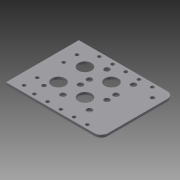
# Autodesk Inventor part: talon plate short
Saved by Autodesk Inventor 2015 (Build 190159000, 159)
## iProperties
Created: 2015-02-10
Part Number: talon plate short
Material: Generic
Document SubType Name: Modeling
Designer: sspriggs
Density: 1 g/cm^3
Appearance: Default
Mass: 12.6589 g
Surface Area: 128.442 cm^2
Volume: 12.6589 cm^3
Author: sspriggs
Autodesk Inventor part; units mm, degrees
ref_plane "YZ Plane" through (0, 0, 0) normal (1, 0, 0) x (0, 1, 0)
ref_plane "XZ Plane" through (0, 0, 0) normal (0, 1, 0) x (-1, 0, 0)
ref_plane "Work Plane1" through (-2.7575, 14.1676, 33.7809) normal (0, 1, 0) x (1, 0, 0)
sketch "Sketch1" plane through (-2.7575, 14.1676, 33.7809) normal (0, 1, 0) x (1, 0, 0)
  line L0 (-6.2522, -27.7336) -> (82.6478, -27.7336)
  line L1 (82.6478, -27.7336) -> (82.6478, -97.5836)
  line L2 (82.6478, -97.5836) -> (-6.2522, -97.5836)
  line L3 (-6.2522, -97.5836) -> (-6.2522, -27.7336)
  point P0 (2.7575, 33.7809)
  dimension "d0" = 69.85
  dimension "d1" = 88.9
  constraints: 8 end point, 2 parallel, 1 horizontal, 1 perpendicular
  measures "d0" distance of L0.end L1.end
  measures "d1" distance of L1.end L2.end
extrude "Extrusion1" add sketch "Sketch1" along normal blind 2.286
sketch "Sketch2" plane through (-2.7575, 16.4536, 33.7809) normal (0, 1, 0) x (1, 0, 0)
  line L0 (82.6478, -27.7336) -> (-6.2522, -27.7336) projected
  line L1 (-6.2522, -27.7336) -> (-6.2522, -97.5836) projected
  line L2 (-6.2522, -97.5836) -> (82.6478, -97.5836) projected
  line L3 (82.6478, -97.5836) -> (82.6478, -27.7336) projected
  circle A0 centre (5.0092, 73.556) radius 1.6383
  circle A1 centre (5.0092, 60.856) radius 1.6383
  circle A2 centre (5.0092, -2.644) radius 1.6383
  circle A3 centre (5.0092, -78.844) radius 1.6383
  circle A4 centre (5.0092, -91.544) radius 1.6383
  circle A5 centre (5.0092, -40.744) radius 1.6383
  circle A6 centre (5.0092, -53.444) radius 1.6383
  circle A7 centre (5.0092, 10.056) radius 1.6383
  constraints: 8 centre point
extrude "Extrusion2" cut sketch "Sketch2" against normal blind 2.286 contours A0 | A1 | A2 | A3 | A4 | A5 | A6 | A7
sketch "Sketch3" plane through (-2.7575, 16.4536, 33.7809) normal (0, 1, 0) x (1, 0, 0)
  line L0 (82.6478, -97.5836) -> (-6.2522, -97.5836) projected
  line L1 (82.6478, -27.7336) -> (-6.2522, -27.7336) projected
  point P0 (2.7575, 33.7809)
  point P1 (17.1634, -31.5436)
  point P2 (17.1634, -93.7736)
  dimension "d7" = 3.81
  dimension "d8" = 3.81
  constraints: 1 vertical alignment
  measures "d7" distance from line of L0 point (17.163, -93.774)
  measures "d8" distance from line of L1 point (17.163, -31.544)
hole "Hole1" at (14.406, 16.4536, 65.3245) at (14.406, 16.4536, 127.5545) direction (0, -1, 0) diameter 3.2766 depth 2.286 tip angle 118
pattern_linear "Rectangular Pattern1" count 5 spacing 12.7 along (1, 0, 0) of "Hole1"
sketch "Sketch6" plane through (79.8904, 14.1676, 131.3645) normal (1, 0, 0) x (0, 0, -1)
  line L0 (69.85, 2.286) -> (0, 2.286)
  line L1 (0, 2.286) -> (0, 0)
  line L2 (0, 0) -> (69.85, 0)
  line L3 (69.85, 0) -> (69.85, 2.286)
  point P0 (131.3645, -14.1676)
  constraints: 8 end point, 2 parallel, 1 horizontal, 1 perpendicular
extrude "Extrusion4" add sketch "Sketch6" along normal blind 2.286
fillet "Fillet2" radius 6.35 2 edges at (82.1764, 15.3106, 131.3645) (82.1764, 15.3106, 61.5145)
sketch "Sketch7" plane through (-2.7575, 16.4536, 33.7809) normal (0, 1, 0) x (1, 0, 0)
  circle A0 centre (14.7493, -82.094) radius 1.945
  circle A1 centre (76.8777, -40.2856) radius 1.905
  point P0 (2.7575, 33.7809)
  constraints: 2 centre point
extrude "Extrusion5" cut sketch "Sketch7" against normal blind 2.286
sketch "Sketch8" plane through (-2.7575, 16.4536, 33.7809) normal (0, 1, 0) x (1, 0, 0)
  circle A0 centre (18.8172, -46.9734) radius 6.35
  circle A1 centre (31.5172, -38.5914) radius 2.5732
  circle A2 centre (31.5172, -55.3554) radius 2.5732
  point P0 (2.7575, 33.7809)
  dimension "d27" = 12.7
  dimension "d33" = 12.7
  dimension "d34" = 8.382
  dimension "d35" = 8.382
  constraints: 3 centre point, 1 equal radius, 1 vertical alignment
  measures "d27" diameter of A0
  measures "d33" horizontal distance of A1.centre A0.centre
  measures "d34" vertical distance of A0.centre A1.centre
  measures "d35" vertical distance of A0.centre A2.centre
extrude "Extrusion6" cut sketch "Sketch8" against normal blind 25.4
pattern_linear "Rectangular Pattern2" count 2 spacing 25.4 along (1, 0, 0) count 2 spacing 25.4 along (0, 0, 1) of "Extrusion6"
equation "\"d8\" = d7"
equation "\"d35\" = d34"
body "Solid1"
